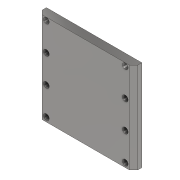
# Autodesk Inventor part: Upper cover of robot head
Saved by Autodesk Inventor 2020.3 (Build 243373010, 373A)
## iProperties
Created: 2021-04-27
Part Number: Upper cover of robot head
Material: Steel, Alloy
Document SubType Name: Modeling
Designer: marti
Density: 7.73 g/cm^3
Appearance: Semi-Polished
Author: marti
Autodesk Inventor part; units mm, degrees
ref_plane "YZ Plane" through (0, 0, 0) normal (1, 0, 0) x (0, 1, 0)
ref_plane "XZ Plane" through (0, 0, 0) normal (0, 1, 0) x (-1, 0, 0)
ref_plane "XY Plane" through (0, 0, 0) normal (0, 0, 1) x (1, 0, 0)
sketch "Sketch1" plane through (0, 0, 0) normal (0, 0, 1) x (1, 0, 0)
  line L0 (0, 0) -> (15, 0)
  arc A0 (-42.9289, -5.4718) -> (-42.9289, -1.7934) centre (-40, -3.6326) ccw
  arc A1 (-42.9289, -38.9718) -> (-42.9289, -35.2934) centre (-40, -37.1326) ccw
  arc A2 (-42.9289, -72.4718) -> (-42.9289, -68.7934) centre (-40, -70.6326) ccw
  arc A3 (-42.9289, -105.9718) -> (-42.9289, -102.2934) centre (-40, -104.1326) ccw
  arc A4 (57.9289, -102.2934) -> (57.9289, -105.9718) centre (55, -104.1326) ccw
  arc A5 (57.9289, -68.7934) -> (57.9289, -72.4718) centre (55, -70.6326) ccw
  arc A6 (57.9289, -35.2934) -> (57.9289, -38.9718) centre (55, -37.1326) ccw
  arc A7 (57.9289, -1.7934) -> (57.9289, -5.4718) centre (55, -3.6326) ccw
  line L1 (0, 0) -> (15, 0)
  spline S0 degree 3 poles (-42.9289, -5.4718) (-43.0252, -5.3184) (-43.1102, -5.1562) (-43.3669, -4.5537) (-43.4585, -4.079) (-43.4585, -3.1862) (-43.3669, -2.7114) (-43.1102, -2.109) (-43.0252, -1.9468) (-42.9289, -1.7934) knots 1.816211 1.816211 1.816211 1.816211 1.867954 1.867954 2.001868 2.001868 2.135782 2.135782 2.187525 2.187525 2.187525 2.187525
  spline S1 degree 3 poles (-42.9289, -105.9718) (-43.0252, -105.8184) (-43.1102, -105.6562) (-43.3669, -105.0537) (-43.4585, -104.579) (-43.4585, -103.6862) (-43.3669, -103.2114) (-43.1102, -102.609) (-43.0252, -102.4468) (-42.9289, -102.2934) knots 1.816211 1.816211 1.816211 1.816211 1.867954 1.867954 2.001868 2.001868 2.135782 2.135782 2.187525 2.187525 2.187525 2.187525
  spline S2 degree 3 poles (-42.9289, -72.4718) (-43.0252, -72.3184) (-43.1102, -72.1562) (-43.3669, -71.5537) (-43.4585, -71.079) (-43.4585, -70.1862) (-43.3669, -69.7114) (-43.1102, -69.109) (-43.0252, -68.9468) (-42.9289, -68.7934) knots 1.816211 1.816211 1.816211 1.816211 1.867954 1.867954 2.001868 2.001868 2.135782 2.135782 2.187525 2.187525 2.187525 2.187525
  spline S3 degree 3 poles (-42.9289, -38.9718) (-43.0252, -38.8184) (-43.1102, -38.6562) (-43.3669, -38.0537) (-43.4585, -37.579) (-43.4585, -36.6862) (-43.3669, -36.2114) (-43.1102, -35.609) (-43.0252, -35.4468) (-42.9289, -35.2934) knots 1.816211 1.816211 1.816211 1.816211 1.867954 1.867954 2.001868 2.001868 2.135782 2.135782 2.187525 2.187525 2.187525 2.187525
  arc A8 (57.9289, -38.9718) -> (57.9289, -35.2934) centre (55, -37.1326) ccw
  arc A9 (57.9289, -5.4718) -> (57.9289, -1.7934) centre (55, -3.6326) ccw
  arc A10 (57.9289, -72.4718) -> (57.9289, -68.7934) centre (55, -70.6326) ccw
  arc A11 (57.9289, -105.9718) -> (57.9289, -102.2934) centre (55, -104.1326) ccw
  line L2 (-50, 0.0004) -> (65, 0.0004)
  line L3 (65, 0.0004) -> (65, -109.3496)
  line L4 (65, -109.3496) -> (-50, -109.3496)
  line L5 (-50, -109.3496) -> (-50, 0.0004)
  point P0 (7.5, -111.1326)
  point P1 (84.0033, -110.1193)
  point P2 (84.0033, -111.5873)
  point P3 (-42.9289, -102.2934)
  point P4 (84.0033, -151.6974)
  point P5 (84.0033, -136.8593)
  point P6 (84.0033, -138.3274)
  point P7 (84.0033, -123.4893)
  point P8 (84.0033, -124.9573)
  point P9 (7.5, -109.3496)
  point P10 (-42.9289, -35.2934)
  dimension "d8" = 115
  dimension "d9" = 109.35
  dimension "d10" = 3.633
  constraints: 25 point on circle, 12 centre point, 12 end point, 3 concentric, 3 horizontal, 2 parallel, 1 midpoint, 1 perpendicular, 1 vertical alignment, 62 other
  measures "d8" distance of L3.end L4.end
  measures "d9" distance of L4.end L2.start
  measures "d10" distance from line of L2 A0.centre
extrude "Extrusion1" add sketch "Sketch1" along normal mid plane 10
chamfer "Chamfer1" distance 5 angle 45 2 edges at (-50, -54.6746, 5) (65, -54.6746, 5)
body "Solid1"
